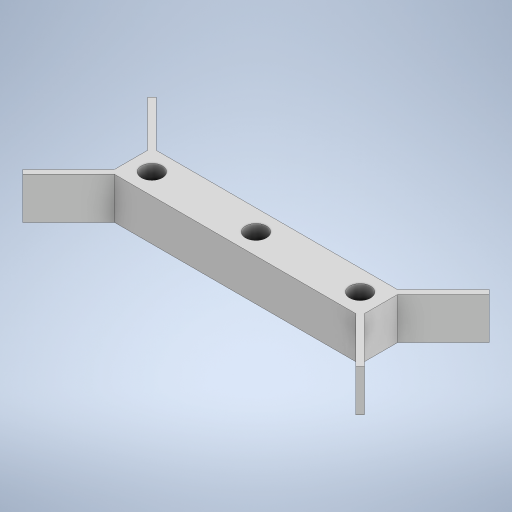
# Autodesk Inventor part: rotational_platform
Saved by Autodesk Inventor 2023.1 (Build 271208000, 208)
## iProperties
Created: 2022-10-07
Part Number: rotational_platform
Material: Generic
Document SubType Name: Modeling
Designer: swang
Density: 1 g/cm^3
Appearance: Default
Author: swang
Autodesk Inventor part; units mm, degrees
ref_plane "YZ Plane" through (0, 0, 0) normal (1, 0, 0) x (0, 1, 0)
ref_plane "XZ Plane" through (0, 0, 0) normal (0, 1, 0) x (-1, 0, 0)
ref_plane "XY Plane" through (0, 0, 0) normal (0, 0, 1) x (1, 0, 0)
sketch "Sketch1" plane through (0, 0, 0) normal (0, 1, 0) x (-1, 0, 0)
  line L0 (-300, 50) -> (300, 50)
  line L1 (300, 50) -> (300, -50)
  line L2 (300, -50) -> (-300, -50)
  line L3 (-300, -50) -> (-300, 50)
  line L4 (-300, 50) -> (300, -50) construction
  line L5 (300, 50) -> (-300, -50) construction
  point P0 (0, 0)
  dimension "d0" = 100
  dimension "d1" = 600
  constraints: 12 end point, 2 midpoint, 2 parallel, 1 horizontal, 1 perpendicular
  measures "d0" distance of L2.end L0.start
  measures "d1" distance of L1.end L2.end
extrude "Extrusion1" add sketch "Sketch1" along normal blind 100
sketch "Sketch2" plane through (0, 100, 0) normal (0, 1, 0) x (1, 0, 0)
  line L0 (300, 50) -> (-300, 50) projected
  line L1 (-300, 50) -> (-400, 150) construction
  line L2 (-410.2193, 150) -> (-300, 39.7807)
  line L3 (-300, 39.7807) -> (-289.7807, 50)
  line L4 (-289.7807, 50) -> (-400, 160.2193)
  line L5 (-400, 160.2193) -> (-410.2193, 150)
  line L6 (-410.2193, 150) -> (-289.7807, 50) construction
  line L7 (-300, 39.7807) -> (-400, 160.2193) construction
  point P0 (0, 0)
  point P1 (-350, 100)
  dimension "d4" = 135
  dimension "d5" = 100
  dimension "d6" = 135
  constraints: 14 end point, 3 midpoint, 2 parallel, 1 perpendicular, 1 point on line
  measures "d4" angle of L0 L1
  measures "d5" horizontal distance of L0.end L1.end
  measures "d6" angle of L0 L4
extrude "Extrusion2" add sketch "Sketch2" against normal up to surface (100 mm away)
mirror "Mirror1" about plane through (0, 0, 0) normal (1, 0, 0) of "Extrusion2"
mirror "Mirror2" about plane through (0, 0, 0) normal (0, 0, 1) of "Extrusion2", "Mirror1"
sketch "Sketch4" plane through (0, 100, 0) normal (0, 1, 0) x (1, 0, 0)
  circle A0 centre (0, 0) radius 25
  line L0 (-300, 39.7807) -> (-300, -39.7807) construction
  line L1 (-300, 0) -> (300, 0) construction
  line L2 (300, -39.7807) -> (300, 39.7807) construction
  circle A1 centre (250, 0) radius 25
  line L3 (-50, 0) -> (550, 0) construction
  circle A2 centre (-250, 0) radius 25
  line L4 (-550, 0) -> (50, 0) construction
  circle A3 centre (0, 0) radius 25
  line L5 (-300, 0) -> (300, 0) construction
  dimension "d9" = 50
  dimension "d12" = 250
  dimension "d15" = 250
  constraints: 8 end point, 4 centre point, 2 collinear, 2 horizontal, 2 midpoint, 1 coincident, 13 other
  measures "d9" diameter of A0
  measures "d12" distance of A0.centre A1.centre
  measures "d15" distance of A0.centre A2.centre
extrude "Extrusion3" cut sketch "Sketch4" against normal blind 50
body "Solid1"
